Testsuspension (Autodesk Fusion 360 design; units mm, degrees)
Autodesk Fusion 360 part; units mm, degrees
sketch "Sketch1" plane through (0, 0, 0) normal (0, 0, 1) x (1, 0, 0)
  line L0 (20, -20) -> (-20, -20)
  line L1 (-20, -20) -> (-20, 20)
  line L2 (-20, 20) -> (20, 20)
  line L3 (20, 20) -> (20, -20)
  line L4 (20, -20) -> (-20, 20) construction
  line L5 (-20, -20) -> (20, 20) construction
  line L6 (12.5, -12.5) -> (-12.5, -12.5) construction
  line L7 (-12.5, -12.5) -> (-12.5, 12.5) construction
  line L8 (-12.5, 12.5) -> (12.5, 12.5) construction
  line L9 (12.5, 12.5) -> (12.5, -12.5) construction
  line L10 (12.5, -12.5) -> (-12.5, 12.5) construction
  line L11 (-12.5, -12.5) -> (12.5, 12.5) construction
  circle A0 centre (-12.5, 12.5) radius 2.25
  circle A1 centre (12.5, 12.5) radius 2.25
  circle A2 centre (12.5, -12.5) radius 2.25
  circle A3 centre (-12.5, -12.5) radius 2.25
  dimension "d1" = 40
  dimension "d2" = 40
  dimension "d3" = 25
  dimension "d4" = 25
  dimension "d5" = 4.5
  dimension "d6" = 4.5
  dimension "d7" = 4.5
  dimension "d8" = 4.5
  constraint perpendicular L0 L1
  constraint parallel L0 L2
  constraint parallel L1 L3
  constraint horizontal L0
  constraint coincident L4 origin
  constraint coincident L5 origin
  constraint perpendicular L6 L7
  constraint parallel L6 L8
  constraint parallel L7 L9
  constraint horizontal L6
  constraint coincident L10 origin
  constraint coincident L11 origin
  constraint coincident L7.end L8.start
  constraint coincident L8.end L9.start
  constraint coincident L6.start L9.end
  constraint coincident L6.end L7.start
  measures "d1" distance of L0.end L1.end
  measures "d2" distance of L1.end L2.end
  measures "d3" distance of L7.end L8.end
  measures "d4" distance of L6.end L7.end
  measures "d5" diameter of A0
  measures "d6" diameter of A1
  measures "d7" diameter of A2
  measures "d8" diameter of A3
extrude "Extrude1" add sketch "Sketch1" along normal blind 4
sketch "Sketch2" plane through (0, 0, 4) normal (0, 0, 1) x (-1, 0, 0)
  circle A0 centre (12.5, 12.5) radius 2.25
  circle A1 centre (12.5, -12.5) radius 2.25
  circle A2 centre (-12.5, -12.5) radius 2.25
  circle A3 centre (-12.5, 12.5) radius 2.25
  line L0 (-20, -20) -> (20, -20)
  line L1 (20, -20) -> (20, 20)
  line L2 (20, 20) -> (-20, 20)
  line L3 (-20, 20) -> (-20, -20)
  circle A4 centre (0, 0) radius 10.3
  circle A5 centre (0, 0) radius 12.3
  dimension "d11" = 20.6
  dimension "d12" = 2
  constraint coincident A4.centre A5.centre
  measures "d11" diameter of A4
extrude "Extrude2" add sketch "Sketch2" along normal blind 30 contours A5
sketch "Sketch3" plane through (0, 0, 0) normal (1, 0, 0) x (0, 1, 0)
  line L0 (12.3, 34) -> (-12.3, 34)
  line L1 (-12.3, 4) -> (12.3, 4)
  line L2 (-12.3, 34) -> (12.3, 4) construction
  circle A0 centre (0, 19) radius 2.1
  dimension "d15" = 4.2
  constraint coincident L0.end L2.start
  constraint coincident L1.end L2.end
  constraint midpoint L2 A0.centre
  measures "d15" diameter of A0
extrude "Extrude3" cut sketch "Sketch3" along normal through all and the other way through all
fillet "Fillet1" radius 2 1 edges at (11.4676, -4.4479, 4)
named bodies: "Test_Suspension"
